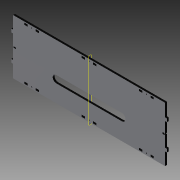
# Autodesk Inventor part: TOP PLATE
Saved by Autodesk Inventor 2013 (Build 170138000, 138)
## iProperties
Created: 2014-06-21
Part Number: TOP PLATE
Material: Generic
Document SubType Name: Modeling
Designer: employee
Density: 1 g/cm^3
Author: employee
Autodesk Inventor part; units mm, degrees
ref_plane "YZ Plane" through (0, 0, 0) normal (1, 0, 0) x (0, 1, 0)
ref_plane "XZ Plane" through (0, 0, 0) normal (0, 1, 0) x (-1, 0, 0)
ref_plane "XY Plane" through (0, 0, 0) normal (0, 0, 1) x (1, 0, 0)
sketch "Sketch1" plane through (0, 0, 0) normal (0, 0, 1) x (1, 0, 0)
  line L0 (463, 164.43) -> (0, 164.43)
  line L1 (0, 164.43) -> (0, -3)
  line L2 (0, -3) -> (463, -3)
  line L3 (463, -3) -> (463, 164.43)
  point P0 (0, 0)
  point P1 (463, 161.43)
  dimension "d0" = 3
  dimension "d1" = 3
  constraints: 8 end point, 2 parallel, 2 point on line, 1 horizontal, 1 perpendicular, 1 other
  measures "d0" distance from line of L2 point (0, 0)
  measures "d1" distance from line of L0 point (463, 161.43)
extrude "Extrusion1" add sketch "Sketch1" along normal blind 5.715
sketch "Sketch2" plane through (0, 0, 5.715) normal (0, 0, 1) x (1, 0, 0)
  line L0 (463, 164.43) -> (0, 164.43) projected
  line L1 (0, 164.43) -> (0, -3) projected
  line L2 (0, -3) -> (463, -3) projected
  line L3 (463, -3) -> (463, 164.43) projected
  line L4 (44, 0) -> (34, 0) projected
  line L5 (44, 5.715) -> (44, 0) projected
  line L6 (34, 5.715) -> (44, 5.715) projected
  line L7 (34, 5.715) -> (34, 0) projected
  line L8 (79, 0) -> (69, 0) projected
  line L9 (79, 5.715) -> (79, 0) projected
  line L10 (69, 5.715) -> (79, 5.715) projected
  line L11 (69, 5.715) -> (69, 0) projected
  line L12 (219, 0) -> (209, 0) projected
  line L13 (219, 5.715) -> (219, 0) projected
  line L14 (209, 5.715) -> (219, 5.715) projected
  line L15 (209, 5.715) -> (209, 0) projected
  line L16 (254, 0) -> (244, 0) projected
  line L17 (254, 5.715) -> (254, 0) projected
  line L18 (244, 5.715) -> (254, 5.715) projected
  line L19 (244, 5.715) -> (244, 0) projected
  line L20 (394, 0) -> (384, 0) projected
  line L21 (394, 5.715) -> (394, 0) projected
  line L22 (384, 5.715) -> (394, 5.715) projected
  line L23 (384, 5.715) -> (384, 0) projected
  line L24 (429, 0) -> (419, 0) projected
  line L25 (429, 5.715) -> (429, 0) projected
  line L26 (419, 5.715) -> (429, 5.715) projected
  line L27 (419, 5.715) -> (419, 0) projected
  line L28 (429, 155.715) -> (419, 155.715) projected
  line L29 (429, 161.43) -> (429, 155.715) projected
  line L30 (419, 161.43) -> (429, 161.43) projected
  line L31 (419, 161.43) -> (419, 155.715) projected
  line L32 (394, 155.715) -> (384, 155.715) projected
  line L33 (394, 161.43) -> (394, 155.715) projected
  line L34 (384, 161.43) -> (394, 161.43) projected
  line L35 (384, 161.43) -> (384, 155.715) projected
  line L36 (254, 155.715) -> (244, 155.715) projected
  line L37 (254, 161.43) -> (254, 155.715) projected
  line L38 (244, 161.43) -> (254, 161.43) projected
  line L39 (244, 161.43) -> (244, 155.715) projected
  line L40 (219, 155.715) -> (209, 155.715) projected
  line L41 (219, 161.43) -> (219, 155.715) projected
  line L42 (209, 161.43) -> (219, 161.43) projected
  line L43 (209, 161.43) -> (209, 155.715) projected
  line L44 (79, 155.715) -> (69, 155.715) projected
  line L45 (79, 161.43) -> (79, 155.715) projected
  line L46 (69, 161.43) -> (79, 161.43) projected
  line L47 (69, 161.43) -> (69, 155.715) projected
  line L48 (44, 155.715) -> (34, 155.715) projected
  line L49 (44, 161.43) -> (44, 155.715) projected
  line L50 (34, 161.43) -> (44, 161.43) projected
  line L51 (34, 161.43) -> (34, 155.715) projected
  point P0 (0, 0)
extrude "Extrusion2" cut sketch "Sketch2" against normal through all keep common part
sketch "Sketch3" plane through (0, 0, 5.715) normal (0, 0, 1) x (1, 0, 0)
  line L0 (44, 155.715) -> (44, 161.43) projected
  line L1 (69, 161.43) -> (69, 155.715) projected
  line L2 (219, 155.715) -> (219, 161.43) projected
  line L3 (244, 161.43) -> (244, 155.715) projected
  line L4 (394, 155.715) -> (394, 161.43) projected
  line L5 (419, 161.43) -> (419, 155.715) projected
  line L6 (419, 5.715) -> (419, 0) projected
  line L7 (394, 0) -> (394, 5.715) projected
  line L8 (244, 5.715) -> (244, 0) projected
  line L9 (219, 0) -> (219, 5.715) projected
  line L10 (69, 5.715) -> (69, 0) projected
  line L11 (44, 0) -> (44, 5.715) projected
  line L12 (44, 158.5725) -> (69, 158.5725) construction
  circle A0 centre (56.5, 158.5725) radius 1.5
  line L13 (219, 158.5725) -> (244, 158.5725) construction
  circle A1 centre (231.5, 158.5725) radius 1.5
  line L14 (394, 158.5725) -> (419, 158.5725) construction
  circle A2 centre (406.5, 158.5725) radius 1.5
  line L15 (44, 2.8575) -> (69, 2.8575) construction
  circle A3 centre (56.5, 2.8575) radius 1.5
  line L16 (219, 2.8575) -> (244, 2.8575) construction
  circle A4 centre (231.5, 2.8575) radius 1.5
  line L17 (394, 2.8575) -> (419, 2.8575) construction
  circle A5 centre (406.5, 2.8575) radius 1.5
  point P0 (0, 0)
  dimension "d6" = 3
  dimension "d8" = 3
  dimension "d9" = 3
  dimension "d10" = 3
  dimension "d11" = 3
  dimension "d12" = 3
  constraints: 22 midpoint, 12 end point, 6 centre point
  measures "d6" diameter of A0
  measures "d8" diameter of A1
  measures "d9" diameter of A2
  measures "d10" diameter of A3
  measures "d11" diameter of A4
  measures "d12" diameter of A5
extrude "Extrusion3" cut sketch "Sketch3" against normal through all
sketch "Sketch4" plane through (0, 0, 5.715) normal (0, 0, 1) x (1, 0, 0)
  line L0 (0, 164.43) -> (0, -3) projected
  line L1 (0, 82.215) -> (8.285, 82.215)
  line L2 (8.285, 82.215) -> (8.285, 79.215)
  line L3 (8.285, 79.215) -> (0, 79.215)
  line L4 (0, 79.215) -> (0, 82.215)
  line L5 (4.285, 83.465) -> (6.285, 83.465)
  line L6 (6.285, 83.465) -> (6.285, 77.965)
  line L7 (6.285, 77.965) -> (4.285, 77.965)
  line L8 (4.285, 77.965) -> (4.285, 83.465)
  point P0 (0, 0)
  point P1 (0, 80.715)
  point P2 (6.285, 80.715)
  point P3 (8.285, 80.715)
  dimension "d15" = 3
  dimension "d17" = 5.5
  dimension "d18" = 6.285
  dimension "d19" = 2
  dimension "d20" = 8.285
  constraints: 16 end point, 4 midpoint, 4 parallel, 2 horizontal, 2 perpendicular, 1 horizontal alignment, 1 point on line
  measures "d15" distance of L1.end L2.end
  measures "d17" distance of L5.end L6.end
  measures "d18" distance between parallel lines of L6 L0
  measures "d19" distance of L5.start L5.end
  measures "d20" distance from line of point (8.285, 80.715) L0
extrude "Extrusion4" cut sketch "Sketch4" against normal through all
ref_plane "Work Plane1" through (231.5, 164.43, 0) normal (-1, 0, 0) x (0, 0, 1)
sketch "Sketch5" plane through (0, 0, 5.715) normal (0, 0, 1) x (1, 0, 0)
  line L0 (0, 79.215) -> (0, -3) projected
  line L1 (0, 164.43) -> (0, 82.215) projected
  line L2 (8.285, 82.215) -> (8.285, 79.215) projected
  line L3 (0, 125.715) -> (-5.715, 125.715)
  line L4 (-5.715, 125.715) -> (-5.715, 115.715)
  line L5 (-5.715, 115.715) -> (0, 115.715)
  line L6 (0, 115.715) -> (0, 125.715)
  line L7 (0, 45.715) -> (-5.715, 45.715)
  line L8 (-5.715, 45.715) -> (-5.715, 35.715)
  line L9 (-5.715, 35.715) -> (0, 35.715)
  line L10 (0, 35.715) -> (0, 45.715)
  line L11 (-5.715, 45.715) -> (-5.715, 115.715)
  point P0 (0, 0)
  point P1 (8.285, 80.715)
  point P2 (-5.715, 80.715)
  point P3 (8.285, 80.715)
  dimension "d23" = 35
  dimension "d26" = 5.715
  dimension "d27" = 10
  constraints: 18 end point, 5 parallel, 3 midpoint, 2 horizontal, 2 perpendicular, 2 point on line, 1 collinear, 1 horizontal alignment
  measures "d23" distance from line of L7 point (8.285, 80.715)
  measures "d26" distance of L7.start L7.end
  measures "d27" distance of L7.end L8.end
extrude "Extrusion5" add sketch "Sketch5" against normal up to surface (5.715 mm away)
mirror "Mirror1" about plane through (231.5, 164.43, 0) normal (-1, 0, 0) of "Extrusion5", "Extrusion4"
sketch "Sketch6" plane through (0, 0, 5.715) normal (0, 0, 1) x (1, 0, 0)
  circle A0 centre (231.5, 2.8575) radius 1.5 projected
  line L0 (356, 95.715) -> (341, 95.715) projected
  line L1 (341, 25.715) -> (356, 25.715) projected
  line L2 (348.5, 25.715) -> (348.5, 95.715)
  line L3 (331.5, 49.715) -> (131.5, 49.715)
  arc A1 (131.5, 71.715) -> (131.5, 49.715) centre (131.5, 60.715) ccw
  line L4 (131.5, 71.715) -> (331.5, 71.715)
  arc A2 (331.5, 49.715) -> (331.5, 71.715) centre (331.5, 60.715) ccw
  point P0 (0, 0)
  point P1 (231.5, 49.715)
  point P2 (348.5, 60.715)
  dimension "d30" = 200
  dimension "d32" = 22
  constraints: 6 end point, 4 midpoint, 4 point on circle, 4 tangent, 2 centre point, 1 horizontal alignment, 1 parallel, 1 perpendicular, 1 vertical alignment
  measures "d30" distance of A1.centre A2.centre
  measures "d32" distance between parallel lines of L3 L4
extrude "Extrusion6" cut sketch "Sketch6" against normal through all contours L3 A1 L4 A2
body "Solid1"
